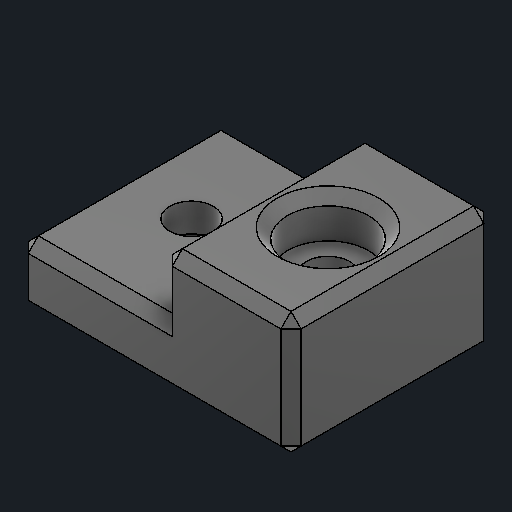
# Autodesk Inventor part: Part2
Saved by Autodesk Inventor 2026.2 (Build 302298000, 298)
## iProperties
Created: 2026-07-19
Part Number: Part2
Material: ABS Plastic
Document SubType Name: Modeling
Designer: JoshuaEah
Density: 1.06 g/cm^3
Appearance: Smooth - Black
Author: JoshuaEah
Autodesk Inventor part; units mm, degrees
ref_plane "YZ Plane" through (0, 0, 0) normal (1, 0, 0) x (0, 1, 0)
ref_plane "XZ Plane" through (0, 0, 0) normal (0, 1, 0) x (-1, 0, 0)
ref_plane "XY Plane" through (0, 0, 0) normal (0, 0, 1) x (1, 0, 0)
sketch "Base Sketch" plane through (0, 0, 0) normal (0, 1, 0) x (-1, 0, 0)
  line L0 (0, 0) -> (-26.9, 0)
  line L1 (-26.9, 0) -> (-26.9, -20)
  line L2 (-26.9, -20) -> (0, -20)
  line L3 (0, -20) -> (0, 0)
  line L4 (-14.2, -20) -> (-14.2, 0)
  line L5 (-10.6, -7.9793) -> (-7.1, -5.9585)
  line L6 (-7.1, -5.9585) -> (-3.6, -7.9793)
  line L7 (-3.6, -7.9793) -> (-3.6, -12.0207)
  line L8 (-3.6, -12.0207) -> (-7.1, -14.0415)
  line L9 (-7.1, -14.0415) -> (-10.6, -12.0207)
  line L10 (-10.6, -12.0207) -> (-10.6, -7.9793)
  point P0 (-20.55, -10)
  point P1 (-26.9, -10)
  point P2 (-7.1, -10)
  point P3 (0, -10)
  point P4 (-7.1, -10)
  dimension "d0" = 20
  dimension "d5" = 14.2
  dimension "d7" = 6.35
  dimension "d8" = 6.35
  dimension "d25" = 7.1
  dimension "d36" = 7
  constraints: 22 end point, 2 coincident, 2 horizontal alignment, 2 midpoint, 2 parallel, 2 perpendicular, 2 point on line, 1 horizontal, 1 vertical, 13 other
  measures "d0" distance of L2.end L0.start
  measures "d5" distance between parallel lines of L4 L3
  measures "d7" distance from line of L4 point (-20.55, -10)
  measures "d8" distance from line of L1 point (-20.55, -10)
  measures "d25" distance from line of L3 point (-7.1, -10)
  measures "d36" distance between parallel lines of L6 L9
extrude "BasePlate" add sketch "Base Sketch" against normal blind 6 contours L3 L2 L4 L0 | L4 L2 L1 L0 | L5 L6 L7 L8 L9 L10
hole "Load Screw Hole" at (7.1, 0, -10) direction (0, -1, 0) diameter 4.2926 end through all clearance for "Socket Head Cap Screw" size "M4" standard "Ansi Metric M Profile"
extrude "Top Section" add sketch "Base Sketch" along normal blind 6 contours L4 L2 L1 L0
sketch "Sketch2" plane through (0, 6, 0) normal (0, 1, 0) x (1, 0, 0)
  point P0 (20.55, 10)
hole "Extrusion Mount Screw" at (20.55, 6, -10) direction (0, -1, 0) diameter 4.2926 end through all counterbore diameter 8.001 counterbore depth 3.9878 clearance for "Socket Head Cap Screw" size "M4" standard "Ansi Metric M Profile"
chamfer "Chamfer" distance 1 angle 45 18 edges at (7.1, 0, -20) (14.2, 3, -20) (20.55, 6, -20) (26.9, 6, -10) (20.55, 6, 0) (14.2, 3, 0) (7.1, 0, 0) (0, -3, 0) (26.9, 0, 0) (26.9, 0, -20) (13.45, -6, -20) (26.9, -6, -10) (13.45, -6, 0) (0, -6, -10) (0, -3, -20) (0, 0, -10) (14.2, 6, -10) (20.55, 6, -14.0005)
extrude "Hex Nut Slot" cut sketch "Base Sketch" along normal blind 3.2 from surface at -6 contours L5 L6 L7 L8 L9 L10
thicken "Nut Fit Clearance" operation cut thickness 0.1 both sides no extend neighbours yes toward (-0.5, 0, 0.8660254) faces at (4.7667, -4.9333, -7.3057) (3.6, -4.9333, -10.6736) (5.9333, -4.9333, -13.3679) (9.4333, -4.9333, -12.6943) (10.6, -4.9333, -9.3264) (8.2667, -4.9333, -6.6321)
equation "\"d8\" = d7"
equation "\"d25\" = 0.5 * d5"
equation "\"d9\" = baseThickness"
equation "\"d22\" = chamferSize"
equation "\"baseThickness\" = 6"
equation "\"jawTravel\" = 3"
equation "\"M4_clearance_hole\" = 4.2"
equation "\"slotLength\" = M4_clearance_hole + jawTravel"
equation "\"chamferSize\" = 1"
body "Solid1"
